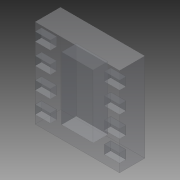
# Autodesk Inventor part: BH1745NUC
Saved by Autodesk Inventor 2013 (Build 170138000, 138)
## iProperties
Created: 2015-06-30
Part Number: BH1745NUC
Material: Ogólny
Document SubType Name: Modeling
Designer: terg
Density: 1 g/cm^3
Author: terg
Autodesk Inventor part; units mm, degrees
ref_plane "YZ Plane" through (0, 0, 0) normal (1, 0, 0) x (0, 1, 0)
ref_plane "XZ Plane" through (0, 0, 0) normal (0, 1, 0) x (-1, 0, 0)
ref_plane "XY Plane" through (0, 0, 0) normal (0, 0, 1) x (1, 0, 0)
sketch "Szkic1" plane through (0, 0, 0) normal (0, 1, 0) x (-1, 0, 0)
  line L0 (0, 0) -> (2, 0)
  line L1 (2, 0) -> (2, 2.1)
  line L2 (2, 2.1) -> (0, 2.1)
  line L3 (0, 2.1) -> (0, 0)
  dimension "d0" = 2
  dimension "d1" = 2.1
  constraints: 8 end point, 2 parallel, 1 horizontal, 1 perpendicular
  measures "d0" distance of L2.end L1.end
  measures "d1" distance of L1.end L0.end
extrude "Wyciągnięcie proste1" add sketch "Szkic1" along normal blind 0.6
sketch "Szkic2" plane through (0, 0, 0) normal (0, -1, 0) x (1, 0, 0)
  line L0 (0, 0) -> (-2, 0) projected
  line L1 (0, 2.1) -> (0, 0) projected
  line L2 (-2, 2.1) -> (0, 2.1) projected
  line L3 (-2, 0) -> (-2, 2.1) projected
  line L4 (0, 0.195) -> (-0.36, 0.195)
  line L5 (-0.36, 0.195) -> (-0.36, 0.405)
  line L6 (-0.36, 0.405) -> (0, 0.405)
  line L7 (0, 0.405) -> (0, 0.195)
  line L8 (0, 0.695) -> (-0.36, 0.695)
  line L9 (-0.36, 0.695) -> (-0.36, 0.905)
  line L10 (-0.36, 0.905) -> (0, 0.905)
  line L11 (0, 0.905) -> (0, 0.695)
  line L12 (0, 1.195) -> (-0.36, 1.195)
  line L13 (-0.36, 1.195) -> (-0.36, 1.405)
  line L14 (-0.36, 1.405) -> (0, 1.405)
  line L15 (0, 1.405) -> (0, 1.195)
  line L16 (0, 1.695) -> (-0.36, 1.695)
  line L17 (-0.36, 1.695) -> (-0.36, 1.905)
  line L18 (-0.36, 1.905) -> (0, 1.905)
  line L19 (0, 1.905) -> (0, 1.695)
  line L20 (-1.64, 0.195) -> (-2, 0.195)
  line L21 (-2, 0.195) -> (-2, 0.405)
  line L22 (-2, 0.405) -> (-1.64, 0.405)
  line L23 (-1.64, 0.405) -> (-1.64, 0.195)
  line L24 (-1.64, 0.695) -> (-2, 0.695)
  line L25 (-2, 0.695) -> (-2, 0.905)
  line L26 (-2, 0.905) -> (-1.64, 0.905)
  line L27 (-1.64, 0.905) -> (-1.64, 0.695)
  line L28 (-1.64, 1.195) -> (-2, 1.195)
  line L29 (-2, 1.195) -> (-2, 1.405)
  line L30 (-2, 1.405) -> (-1.64, 1.405)
  line L31 (-1.64, 1.405) -> (-1.64, 1.195)
  line L32 (-1.64, 1.695) -> (-2, 1.695)
  line L33 (-2, 1.695) -> (-2, 1.905)
  line L34 (-2, 1.905) -> (-1.64, 1.905)
  line L35 (-1.64, 1.905) -> (-1.64, 1.695)
  dimension "d4" = 0.36
  dimension "d5" = 0.21
  dimension "d8" = 0.36
  dimension "d9" = 0.21
  dimension "d10" = 0.36
  dimension "d11" = 0.21
  dimension "d12" = 0.36
  dimension "d13" = 0.21
  dimension "d14" = 0.5
  dimension "d15" = 0.5
  dimension "d16" = 0.5
  dimension "d17" = 0.195
  dimension "d18" = 0.195
  dimension "d19" = 0.36
  dimension "d20" = 0.21
  dimension "d21" = 0.36
  dimension "d22" = 0.36
  dimension "d23" = 0.36
  dimension "d24" = 0.21
  dimension "d25" = 0.21
  dimension "d26" = 0.21
  dimension "d27" = 0.195
  dimension "d28" = 0.5
  dimension "d29" = 0.5
  dimension "d30" = 0.5
  constraints: 64 end point, 16 parallel, 8 horizontal, 8 perpendicular, 8 point on line
  measures "d4" distance of L5.end L6.end
  measures "d5" distance of L4.end L5.end
  measures "d8" distance of L9.end L10.end
  measures "d9" distance of L8.end L9.end
  measures "d10" distance of L13.end L14.end
  measures "d11" distance of L12.end L13.end
  measures "d12" distance of L17.end L18.end
  measures "d13" distance of L16.end L17.end
  measures "d14" distance between parallel lines of L10 L6
  measures "d15" distance between parallel lines of L14 L10
  measures "d16" distance between parallel lines of L18 L14
  measures "d17" distance between parallel lines of L2 L18
  measures "d18" distance between parallel lines of L0 L4
  measures "d19" distance of L21.end L22.end
  measures "d20" distance of L22.end L20.start
  measures "d21" distance of L25.end L26.end
  measures "d22" distance of L29.end L30.end
  measures "d23" distance of L33.end L34.end
  measures "d24" distance of L34.end L32.start
  measures "d25" distance of L30.end L28.start
  measures "d26" distance of L26.end L24.start
  measures "d27" distance between parallel lines of L0 L20
  measures "d28" distance between parallel lines of L26 L22
  measures "d29" distance between parallel lines of L30 L26
  measures "d30" distance between parallel lines of L34 L30
extrude "Wyciągnięcie proste2" cut sketch "Szkic2" against normal blind 0.15 contours L4 L5 L6 L1 | L3 L22 L23 L20 | L8 L9 L10 L1 | L3 L26 L27 L24 | L12 L13 L14 L1 | L3 L30 L31 L28 | L16 L17 L18 L1 | L3 L34 L35 L32
sketch "Szkic3" plane through (0, 0, 0) normal (0, -1, 0) x (1, 0, 0)
  line L0 (-1.64, 0.695) -> (-2, 0.695) projected
  line L1 (-2, 0.405) -> (-1.64, 0.405) projected
  line L2 (-1.64, 0.405) -> (-1.64, 0.195) projected
  line L3 (-1.64, 0.195) -> (-2, 0.195) projected
  line L4 (0, 0.195) -> (-0.36, 0.195) projected
  line L5 (-0.36, 0.195) -> (-0.36, 0.405) projected
  line L6 (-0.36, 0.405) -> (0, 0.405) projected
  line L7 (0, 0.695) -> (-0.36, 0.695) projected
  line L8 (-0.36, 0.695) -> (-0.36, 0.905) projected
  line L9 (-0.36, 0.905) -> (0, 0.905) projected
  line L10 (0, 1.195) -> (0, 0.905) projected
  line L11 (0, 1.195) -> (-0.36, 1.195) projected
  line L12 (-0.36, 1.195) -> (-0.36, 1.405) projected
  line L13 (-0.36, 1.405) -> (0, 1.405) projected
  line L14 (0, 1.695) -> (-0.36, 1.695) projected
  line L15 (-0.36, 1.695) -> (-0.36, 1.905) projected
  line L16 (-0.36, 1.905) -> (0, 1.905) projected
  line L17 (-2, 1.905) -> (-1.64, 1.905) projected
  line L18 (-1.64, 1.905) -> (-1.64, 1.695) projected
  line L19 (-1.64, 1.695) -> (-2, 1.695) projected
  line L20 (-2, 1.405) -> (-1.64, 1.405) projected
  line L21 (-1.64, 1.405) -> (-1.64, 1.195) projected
  line L22 (-1.64, 1.195) -> (-2, 1.195) projected
  line L23 (-2, 0.905) -> (-1.64, 0.905) projected
  line L24 (-1.64, 0.905) -> (-1.64, 0.695) projected
  line L25 (0, 0.2) -> (-0.355, 0.2)
  line L26 (-0.355, 0.2) -> (-0.355, 0.4)
  line L27 (-0.355, 0.4) -> (0, 0.4)
  line L28 (0, 0.4) -> (0, 0.2)
  line L29 (0, 0.7) -> (-0.355, 0.7)
  line L30 (-0.355, 0.7) -> (-0.355, 0.9)
  line L31 (-0.355, 0.9) -> (0, 0.9)
  line L32 (0, 0.9) -> (0, 0.7)
  line L33 (0, 1.2) -> (-0.355, 1.2)
  line L34 (-0.355, 1.2) -> (-0.355, 1.4)
  line L35 (-0.355, 1.4) -> (0, 1.4)
  line L36 (0, 1.4) -> (0, 1.2)
  line L37 (-2, 1.2) -> (-1.645, 1.2)
  line L38 (-1.645, 1.2) -> (-1.645, 1.4)
  line L39 (-1.645, 1.4) -> (-2, 1.4)
  line L40 (-2, 1.4) -> (-2, 1.2)
  line L41 (-2, 0.7) -> (-1.645, 0.7)
  line L42 (-1.645, 0.7) -> (-1.645, 0.9)
  line L43 (-1.645, 0.9) -> (-2, 0.9)
  line L44 (-2, 0.9) -> (-2, 0.7)
  line L45 (-2, 0.2) -> (-1.645, 0.2)
  line L46 (-1.645, 0.2) -> (-1.645, 0.4)
  line L47 (-1.645, 0.4) -> (-2, 0.4)
  line L48 (-2, 0.4) -> (-2, 0.2)
  line L49 (0, 1.7) -> (-0.355, 1.7)
  line L50 (-0.355, 1.7) -> (-0.355, 1.9)
  line L51 (-0.355, 1.9) -> (0, 1.9)
  line L52 (0, 1.9) -> (0, 1.7)
  line L53 (-2, 1.7) -> (-1.645, 1.7)
  line L54 (-1.645, 1.7) -> (-1.645, 1.9)
  line L55 (-1.645, 1.9) -> (-2, 1.9)
  line L56 (-2, 1.9) -> (-2, 1.7)
  dimension "d33" = 0.005
  dimension "d34" = 0.005
  dimension "d35" = 0.005
  dimension "d36" = 0.005
  dimension "d37" = 0.005
  dimension "d38" = 0.005
  dimension "d39" = 0.005
  dimension "d40" = 0.005
  dimension "d41" = 0
  dimension "d42" = 0.005
  dimension "d43" = 0.005
  dimension "d44" = 0.005
  dimension "d45" = 0.005
  dimension "d46" = 0.005
  dimension "d47" = 0.005
  dimension "d48" = 0.005
  dimension "d49" = 0.005
  dimension "d50" = 0.005
  dimension "d51" = 0.005
  dimension "d52" = 0.005
  dimension "d53" = 0.005
  dimension "d54" = 0.005
  dimension "d55" = 0.005
  dimension "d56" = 0.005
  dimension "d57" = 0.005
  constraints: 64 end point, 16 parallel, 8 horizontal, 8 perpendicular
  measures "d33" distance between parallel lines of L4 L25
  measures "d34" distance between parallel lines of L5 L26
  measures "d35" distance between parallel lines of L6 L27
  measures "d36" distance between parallel lines of L7 L29
  measures "d37" distance between parallel lines of L9 L31
  measures "d38" distance between parallel lines of L8 L30
  measures "d39" distance between parallel lines of L12 L34
  measures "d40" distance between parallel lines of L11 L33
  measures "d41" distance between parallel lines of L10 L36
  measures "d42" distance between parallel lines of L13 L35
  measures "d43" distance between parallel lines of L14 L49
  measures "d44" distance between parallel lines of L15 L50
  measures "d45" distance between parallel lines of L16 L51
  measures "d46" distance between parallel lines of L17 L55
  measures "d47" distance between parallel lines of L18 L54
  measures "d48" distance between parallel lines of L19 L53
  measures "d49" distance between parallel lines of L20 L39
  measures "d50" distance between parallel lines of L21 L38
  measures "d51" distance between parallel lines of L22 L37
  measures "d52" distance between parallel lines of L23 L43
  measures "d53" distance between parallel lines of L24 L42
  measures "d54" distance between parallel lines of L0 L41
  measures "d55" distance between parallel lines of L1 L47
  measures "d56" distance between parallel lines of L2 L46
  measures "d57" distance between parallel lines of L3 L45
extrude "Wyciągnięcie proste3" add sketch "Szkic3" against normal blind 0.149
sketch "Szkic4" plane through (0, 0, 0) normal (0, -1, 0) x (1, 0, 0)
  line L0 (0, 0) -> (-2, 0) projected
  line L1 (0, 2.1) -> (0, 1.905) projected
  line L2 (-2, 2.1) -> (0, 2.1) projected
  line L3 (-2, 1.905) -> (-2, 2.1) projected
  line L4 (-1.375, 1.8) -> (-0.625, 1.8)
  line L5 (-0.625, 1.8) -> (-0.625, 0.3)
  line L6 (-0.625, 0.3) -> (-1.375, 0.3)
  line L7 (-1.375, 0.3) -> (-1.375, 1.8)
  dimension "d60" = 0.75
  dimension "d62" = 1.5
  dimension "d63" = 0.3
  dimension "d64" = 0.3
  dimension "d65" = 0.625
  dimension "d66" = 0.625
  constraints: 8 end point, 2 parallel, 1 horizontal, 1 perpendicular
  measures "d60" distance of L4.start L4.end
  measures "d62" distance of L4.end L5.end
  measures "d63" distance between parallel lines of L2 L4
  measures "d64" distance between parallel lines of L0 L6
  measures "d65" distance between parallel lines of L3 L7
  measures "d66" distance between parallel lines of L1 L5
extrude "Wyciągnięcie proste4" cut sketch "Szkic4" against normal blind 0.35
sketch "Szkic5" plane through (0, 0, 0) normal (0, -1, 0) x (1, 0, 0)
  line L0 (-1.375, 0.3) -> (-1.375, 1.8) projected
  line L1 (-1.375, 1.8) -> (-0.625, 1.8) projected
  line L2 (-0.625, 1.8) -> (-0.625, 0.3) projected
  line L3 (-0.625, 0.3) -> (-1.375, 0.3) projected
  line L4 (-1.37, 1.795) -> (-0.63, 1.795)
  line L5 (-0.63, 1.795) -> (-0.63, 0.305)
  line L6 (-0.63, 0.305) -> (-1.37, 0.305)
  line L7 (-1.37, 0.305) -> (-1.37, 1.795)
  dimension "d69" = 0.005
  dimension "d70" = 0.005
  dimension "d71" = 0.005
  dimension "d72" = 0.005
  constraints: 8 end point, 2 parallel, 1 horizontal, 1 perpendicular
  measures "d69" distance between parallel lines of L2 L5
  measures "d70" distance between parallel lines of L0 L7
  measures "d71" distance between parallel lines of L1 L4
  measures "d72" distance between parallel lines of L3 L6
extrude "Wyciągnięcie proste5" add sketch "Szkic5" against normal blind 0.345 contours L4 L5 L6 L7
equation "\"d8\" = d4"
equation "\"d9\" = d5"
equation "\"d10\" = d8"
equation "\"d11\" = d9"
equation "\"d12\" = d10"
equation "\"d13\" = d11"
equation "\"d17\" = d18"
equation "\"d19\" = d4"
equation "\"d20\" = d5"
equation "\"d21\" = d19"
equation "\"d22\" = d21"
equation "\"d23\" = d22"
equation "\"d24\" = d5"
equation "\"d25\" = d5"
equation "\"d26\" = d5"
equation "\"d27\" = d18"
equation "\"d28\" = d14"
equation "\"d29\" = d15"
equation "\"d30\" = d15"
equation "\"d34\" = d33"
equation "\"d35\" = d33"
equation "\"d36\" = d33"
equation "\"d37\" = d33"
equation "\"d38\" = d34"
equation "\"d39\" = d34"
equation "\"d40\" = d33"
equation "\"d42\" = d33"
equation "\"d43\" = d33"
equation "\"d44\" = d34"
equation "\"d45\" = d33"
equation "\"d46\" = d33"
equation "\"d47\" = d34"
equation "\"d48\" = d33"
equation "\"d49\" = d33"
equation "\"d50\" = d34"
equation "\"d51\" = d34"
equation "\"d52\" = d34"
equation "\"d53\" = d33"
equation "\"d54\" = d33"
equation "\"d55\" = d33"
equation "\"d56\" = d33"
equation "\"d57\" = d33"
equation "\"d63\" = d64"
equation "\"d65\" = d66"
equation "\"d70\" = d69"
equation "\"d71\" = d69"
equation "\"d72\" = d69"
